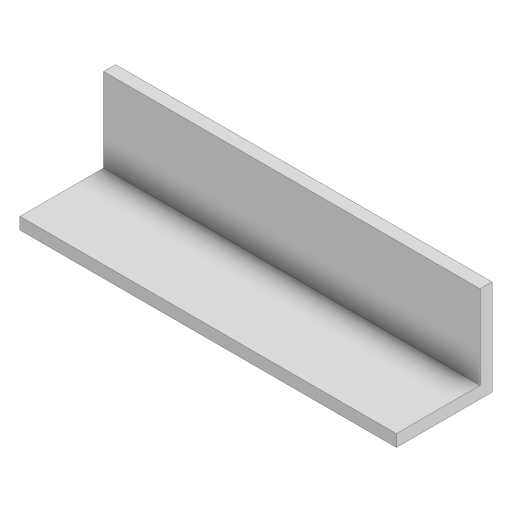
# Autodesk Inventor part: SOPORTE LATERAL DE GUIA CILINDRICA
Saved by Autodesk Inventor 2024 (Build 280153000, 153)
## iProperties
Created: 2024-06-22
Part Number: SOPORTE LATERAL DE GUIA CILINDRICA
Material: Generic
Document SubType Name: Modeling
Designer: Jhuliams
Density: 1 g/cm^3
Appearance: Default
Author: Jhuliams
Autodesk Inventor part; units mm, degrees
ref_plane "YZ Plane" through (0, 0, 0) normal (1, 0, 0) x (0, 1, 0)
ref_plane "XZ Plane" through (0, 0, 0) normal (0, 1, 0) x (-1, 0, 0)
ref_plane "XY Plane" through (0, 0, 0) normal (0, 0, 1) x (1, 0, 0)
sketch "Sketch1" plane through (0, 0, 0) normal (1, 0, 0) x (0, 1, 0)
  line L0 (0, 0) -> (25.4, 0)
  line L1 (25.4, 0) -> (25.4, 3.175)
  line L2 (25.4, 3.175) -> (0, 3.175)
  line L3 (0, 3.175) -> (0, 0)
  line L4 (0, 0) -> (0, 25.4)
  line L5 (0, 25.4) -> (3.175, 25.4)
  line L6 (3.175, 25.4) -> (3.175, 3.175)
  point P0 (3.175, 3.175)
  dimension "d0" = 25.4
  dimension "d1" = 3.175
  dimension "d2" = 25.4
  dimension "d3" = 25.4
  dimension "d4" = 3.175
  dimension "d5" = 90
  constraints: 14 end point, 3 perpendicular, 1 horizontal, 1 vertical
  measures "d0" distance of L0.start L0.end
  measures "d1" distance of L0.end L1.end
  measures "d2" distance of L1.end L2.end
  measures "d3" distance of L0.start L4.end
  measures "d4" distance of L4.end L5.end
  measures "d5" angle of L4 L5
extrude "Extrusion1" add sketch "Sketch1" along normal blind 100
body "Solid1"
